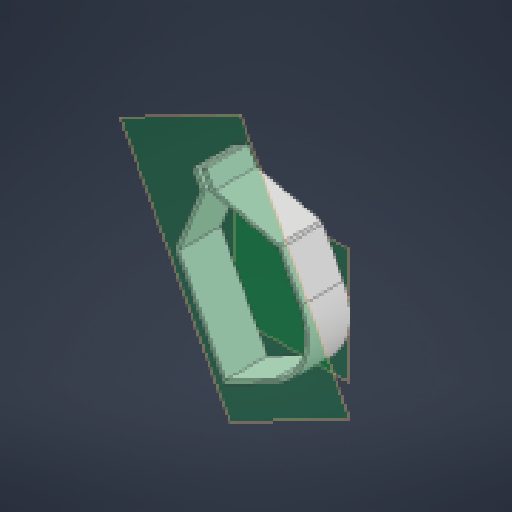
# Autodesk Inventor part: housing_spool
Saved by Autodesk Inventor 2024 (Build 280153000, 153)
## iProperties
Created: 2026-03-24
Part Number: housing_spool
Material: Generic
Document SubType Name: Modeling
Designer: schar
Density: 1 g/cm^3
Appearance: Default
Author: schar
Autodesk Inventor part; units mm, degrees
ref_plane "YZ Plane" through (0, 0, 0) normal (1, 0, 0) x (0, 1, 0)
ref_plane "XZ Plane" through (0, 0, 0) normal (0, 1, 0) x (-1, 0, 0)
ref_plane "XY Plane" through (0, 0, 0) normal (0, 0, 1) x (1, 0, 0)
sketch "Sketch1" plane through (0, 0, 0) normal (0, 0, 1) x (1, 0, 0)
  circle A0 centre (0, 0) radius 30
  line L0 (10.4876, 34.2087) -> (33.8038, -10.3608)
  line L1 (0, 0) -> (41.4605, 21.6898)
  line L2 (0, 0) -> (-43.0442, -22.5183)
  line L3 (-26.5822, -13.9063) -> (-28.3544, -14.8334)
  line L4 (26.5822, 13.9063) -> (28.3544, 14.8334)
  line L5 (8.7104, 28.7647) -> (-22.4507, 46.1509)
  line L6 (-16.4978, 49.2651) -> (10.4876, 34.2087)
  line L7 (-25.1089, 44.7603) -> (-28.5964, 9.2479)
  line L8 (-34.082, 10.8925) -> (-31.0618, 41.6461)
  circle A1 centre (0, 0) radius 32
  circle A2 centre (0, 0) radius 34
  line L9 (15.7605, -30.1265) -> (-26.153, -52.0533)
  line L10 (-30.1265, -15.7605) -> (-6.3352, -61.238)
  line L11 (-30.1265, -15.7605) -> (-49.9852, 22.1997)
  line L12 (-10.7657, -33.6771) -> (-34.082, 10.8925)
  line L13 (10.4876, 34.2087) -> (-34.082, 10.8925)
  line L14 (-34.082, 10.8925) -> (-52.6736, 1.1664)
  line L15 (10.4876, 34.2087) -> (31.4936, 45.1979)
  line L16 (30.1265, 15.7605) -> (13.2261, 48.0659)
  line L17 (28.3544, 14.8334) -> (11.454, 47.1389)
  line L18 (-28.3544, -14.8334) -> (-48.1167, 22.9426)
  line L19 (14.8334, -28.3544) -> (-13.521, -43.1878)
  line L20 (16.5572, 37.384) -> (-22.4507, 46.1509)
  line L21 (-22.4507, 46.1509) -> (-20.6785, 47.078)
  line L22 (16.5572, 37.384) -> (20.2036, 53.6084)
  line L23 (16.5572, 37.384) -> (16.9957, 39.3353)
  line L24 (16.9957, 39.3353) -> (-19.7098, 47.5848)
  line L25 (-19.7098, 47.5848) -> (-20.6785, 47.078)
  line L26 (18.3293, 38.3111) -> (16.9957, 39.3353)
  line L27 (-61.7786, 118.0912) -> (-13.9743, 26.7122)
  line L28 (-42.0046, 8.4697) -> (-27.8498, 43.3264)
  line L29 (-40.1516, 7.7172) -> (-25.1089, 44.7603)
  line L30 (-25.1089, 44.7603) -> (-26.8811, 43.8332)
  line L31 (-27.8498, 43.3264) -> (-26.8811, 43.8332)
  line L32 (-40.1516, 7.7172) -> (-42.0046, 8.4697)
  line L33 (-41.9237, 6.7901) -> (-42.0046, 8.4697)
  line L34 (-40.1516, 7.7172) -> (-55.5588, 13.9738)
  line L35 (-19.7098, 47.5848) -> (-24.3452, 56.4455)
  line L36 (-21.1333, 58.1259) -> (-27.0861, 55.0117)
  line L37 (-22.4507, 46.1509) -> (-27.0861, 55.0117)
  line L38 (-27.0861, 55.0117) -> (-24.3452, 56.4455)
  line L39 (-25.1089, 44.7603) -> (-29.7443, 53.621)
  line L40 (-29.7443, 53.621) -> (-35.6972, 50.5068)
  line L41 (-25.1089, 44.7603) -> (-29.7443, 53.621)
  line L42 (-27.8498, 43.3264) -> (-32.4852, 52.1871)
  line L43 (-29.7443, 53.621) -> (-32.4852, 52.1871)
  line L44 (-13.521, -43.1878) -> (-28.3544, -14.8334)
  line L45 (-61.8482, 118.2241) -> (-14.0438, 26.8451)
  point P0 (8.2214, 9.3684)
  point P1 (-61.7786, 118.0912)
  point P2 (-13.9743, 26.7122)
  point P3 (-14.366, -45.887)
  dimension "d0" = 2
  dimension "d1" = 2
  dimension "d2" = 68
  dimension "d3" = 34
  dimension "d4" = 2
  dimension "d5" = 2
  dimension "d44" = 64
  dimension "d45" = 49.717
  dimension "d46" = 73.507
  dimension "d47" = 7.058
  dimension "d48" = 25.45
  dimension "d49" = 35.85
  dimension "d50" = 25.85
  dimension "d51" = 8.85
  dimension "d52" = 34
  dimension "d53" = 59.15
  dimension "d54" = 12.6858
  dimension "d55" = 11.008
  dimension "d56" = 2.5291
  dimension "d57" = 9.7185
  dimension "d58" = 5.4088
  dimension "d59" = 107.8247
  dimension "d60" = 12.9217
  dimension "d61" = 13.4301
  dimension "d62" = 8.3223
  dimension "d63" = 25.85
  dimension "d64" = 76.7748
  dimension "d65" = 27.2963
  dimension "d66" = 23.2359
  dimension "d67" = 27.4483
  dimension "d68" = 27.4398
  dimension "d69" = 37.885
  dimension "d70" = 55.2569
  dimension "d71" = 57.4671
  dimension "d72" = 11.0758
  dimension "d73" = 75.18
  dimension "d74" = 84.0044
  dimension "d75" = 19.73
  dimension "d76" = -20.9599
  constraints: 90 end point, 14 point on line, 11 parallel, 8 collinear, 7 perpendicular, 7 point on circle, 5 tangent, 3 centre point, 2 coincident, 14 other
  measures "d0" distance of L3.start L18.start
  measures "d1" distance of L4.start L4.end
  measures "d2" diameter of A2
  measures "d3" distance between parallel lines of L2 L9
  measures "d4" distance of L5.end L25.end
  measures "d5" distance of L20.start L23.end
  measures "d44" diameter of A1
  measures "d45" angle of L34 L14
  measures "d46" angle of L32 L8
  measures "d47" angle of L5 L34
  measures "d48" distance between parallel lines of L2 L14
  measures "d49" distance between parallel lines of L43 L14
  measures "d50" distance between parallel lines of L31 L14
  measures "d51" distance between parallel lines of L11 L12
  measures "d52" distance of the line from the sketch origin of L11
  measures "d53" distance between parallel lines of L0 L11
  measures "d54" distance from line of L34.end L14
  measures "d55" distance from line of L14.end L33
  measures "d56" distance from line of L2.end L33
  measures "d57" distance from line of L11.end L34
  measures "d58" distance from line of L18.end L33
  measures "d59" distance from line of point (-61.779, 118.091) L14
  measures "d60" distance from line of L9.end L33
  measures "d61" distance from line of L7.end L33
  measures "d62" distance from line of L40.end L33
  measures "d63" distance from line of L8.end L14
  measures "d64" distance from line of L10.end L14
  measures "d65" distance from line of L12.start L34
  measures "d66" distance from line of L36.start L33
  measures "d67" distance from line of point (-13.974, 26.712) L34
  measures "d68" distance from line of L6.start L33
  measures "d69" distance from line of L5.start L34
  measures "d70" distance from line of L17.end L33
  measures "d71" distance from line of L16.end L32
  measures "d72" distance from line of L0.end L34
  measures "d73" distance from line of L15.end L33
  measures "d74" distance from line of L1.end L33
  measures "d75" distance from line of point (8.221, 9.368) L34
  measures "d76" distance from line of point (8.221, 9.368) L14
ref_plane "Work Plane1" through (0, 0, -14) normal (0, 0, -1) x (-1, 0, 0)
extrude "Extrusion1" add sketch "Sketch1" against normal up to surface (14 mm away) contours L17 A2 L1 | L1 A2 L0 A1 | L0 A2 L19 A1 | A2 L17 L15 L16 | L15 L22 L26 | L20 L6 L24 L17 | L17 L24 L22 | L44 A2 L2 | L2 A2 L18 | L9 L10 A2 L44 L19 | L20 L21 L25 L24 L6 | L11 L14 L18 A2 | L37 L36 L35 L25 L21 | L33 L32 L14 | L32 L28 L18 | L18 L28 L8 L29 | L8 L28 L31 L30 L29 | L30 L31 L42 L40 L39
ref_plane "Work Plane2" through (-8.5115, 15.9463, 10) normal (0, 0, -1) x (-0.886074, -0.4635438, 0)
sketch "Sketch3" plane through (0, 0, 0) normal (0, 0, 1) x (1, 0, 0)
  line L0 (-29.7443, 53.621) -> (-32.4852, 52.1871) projected
  line L1 (-32.4852, 52.1871) -> (-27.8498, 43.3264) projected
  line L2 (-27.8498, 43.3264) -> (-42.0046, 8.4697) projected
  line L3 (-42.0046, 8.4697) -> (-41.9237, 6.7901) projected
  line L4 (-41.9237, 6.7901) -> (-14.366, -45.887) projected
  line L5 (-14.366, -45.887) -> (15.7605, -30.1265) projected
  arc A0 (15.7605, -30.1265) -> (30.1265, 15.7605) centre (0, 0) ccw projected
  line L6 (30.1265, 15.7605) -> (18.3293, 38.3111) projected
  line L7 (18.3293, 38.3111) -> (16.9957, 39.3353) projected
  line L8 (16.9957, 39.3353) -> (-19.7098, 47.5848) projected
  line L9 (-19.7098, 47.5848) -> (-24.3452, 56.4455) projected
  line L10 (-24.3452, 56.4455) -> (-27.0861, 55.0117) projected
  line L11 (-27.0861, 55.0117) -> (-22.4507, 46.1509) projected
  line L12 (-22.4507, 46.1509) -> (16.5572, 37.384) projected
  line L13 (16.5572, 37.384) -> (28.3544, 14.8334) projected
  arc A1 (14.8334, -28.3544) -> (28.3544, 14.8334) centre (0, 0) ccw projected
  line L14 (14.8334, -28.3544) -> (-13.521, -43.1878) projected
  line L15 (-13.521, -43.1878) -> (-40.1516, 7.7172) projected
  line L16 (-40.1516, 7.7172) -> (-25.1089, 44.7603) projected
  line L17 (-25.1089, 44.7603) -> (-29.7443, 53.621) projected
extrude "Extrusion2" add sketch "Sketch3" along normal up to surface (10 mm away)
sketch "Sketch4" plane through (-14.366, -45.887, 10) normal (0, 0, 1) x (0.886074, 0.4635438, 0)
  line L0 (8.7, 9) -> (-10.15, 9) projected
  line L1 (-10.15, 19) -> (-10.15, 9) projected
  line L2 (-10.15, 9) -> (8.7, 9) projected
  line L3 (8.7, 19) -> (8.7, 9) projected
  line L4 (8.7, 19) -> (-10.15, 19) projected
  circle A0 centre (-5.15, 14) radius 2.5 projected
  line L5 (8.7, 59.3) -> (-10.15, 59.3) projected
  line L6 (-10.15, 59.3) -> (-10.15, 49.3) projected
  line L7 (-10.15, 49.3) -> (8.7, 49.3) projected
  line L8 (8.7, 59.3) -> (8.7, 49.3) projected
  circle A1 centre (-5.15, 54.3) radius 2.5 projected
  line L9 (59, 49.3) -> (59, 59.3) projected
  line L10 (59, 49.3) -> (77.85, 49.3) projected
  line L11 (77.85, 49.3) -> (77.85, 59.3) projected
  line L12 (77.85, 59.3) -> (59, 59.3) projected
  circle A2 centre (72.85, 54.3) radius 2.5 projected
  line L13 (59, 9) -> (77.85, 9) projected
  line L14 (77.85, 9) -> (77.85, 19) projected
  line L15 (77.85, 19) -> (59, 19) projected
  line L16 (59, 9) -> (59, 19) projected
  circle A3 centre (72.85, 14) radius 2.5 projected
  line L17 (12.7, 24.85) -> (8.7, 24.85) projected
  line L18 (8.7, 24.85) -> (8.7, 9) projected
  line L19 (8.7, 9) -> (59, 9) projected
  line L20 (59, 9) -> (59, 59.3) projected
  line L21 (59, 59.3) -> (42.0682, 85.15) projected
  line L22 (42.0682, 85.15) -> (42.0682, 95.15) projected
  line L23 (42.0682, 95.15) -> (35.35, 95.15) projected
  line L24 (35.35, 95.15) -> (35.35, 85.15) projected
  line L25 (35.35, 85.15) -> (54.9017, 55.3) projected
  line L26 (54.9017, 55.3) -> (55, 55.3) projected
  line L27 (55, 55.3) -> (55, 13) projected
  line L28 (55, 13) -> (12.7, 13) projected
  line L29 (12.7, 13) -> (12.7, 24.85) projected
  line L30 (77.85, 9) -> (59, 9) projected
  line L31 (59, 9) -> (59, 7) projected
  line L32 (77.85, 7) -> (59, 7) projected
  line L33 (77.85, 9) -> (77.85, 7) projected
  line L34 (8.7, 9) -> (59, 9) projected
  line L35 (8.7, 9) -> (8.7, 7) projected
  line L36 (59, 7) -> (8.7, 7) projected
  line L37 (59, 9) -> (59, 7) projected
  line L38 (59, 19) -> (77.85, 19) projected
  line L39 (77.85, 19) -> (77.85, 21) projected
  line L40 (59, 21) -> (77.85, 21) projected
  line L41 (59, 19) -> (59, 21) projected
  arc A4 (34, 2) -> (66, 34) centre (34, 34) ccw projected
  line L42 (66, 59.45) -> (66, 34) projected
  line L43 (2, 2) -> (2, 59.45) projected
  point P0 (34, 34)
  point P1 (2, 49.3)
  point P2 (2, 59.3)
  point P3 (66, 59.3)
  point P4 (66, 49.3)
  point P5 (62.2666, 19)
  point P6 (53.975, 9)
  point P7 (2, 9)
  point P8 (2, 19)
extrude "Extrusion3" add sketch "Sketch4" against normal blind 3 contours L0 L1 L4 L43 | A4 L16 L19 | L16 A4 L15 L14 L13 | L42 L12 L11 L10 | L43 L7 L6 L5
sketch "Sketch5" plane through (-37.2187, -2.2036, 7) normal (0.4635438, -0.886074, 0) x (0.886074, 0.4635438, 0)
  line L0 (-10.15, 0) -> (0, 0) projected
  line L1 (0, 0) -> (0, -10)
  line L2 (0, -21) -> (0, 3) projected
  line L3 (68, 0) -> (77.85, 0) projected
  line L4 (0, -10) -> (-10.15, 0)
  line L5 (-10.15, 0) -> (68, 0)
  line L6 (68, 0) -> (68, -10)
  line L7 (68, -21) -> (68, 3) projected
  line L8 (68, -10) -> (77.85, 0)
  line L9 (77.85, 3) -> (77.85, 0) projected
  line L10 (-10.15, 3) -> (77.85, 3) projected
  line L11 (-10.15, 3) -> (-10.15, 0) projected
  line L12 (-2.65, 0) -> (-7.65, 0) projected
  point P0 (34, -7)
  dimension "d90" = 10
  dimension "d91" = 10
  constraints: 10 end point, 2 point on line, 1 coincident, 1 horizontal
  measures "d90" distance of L0.end L1.end
  measures "d91" distance of L3.start L6.end
extrude "Extrusion4" add sketch "Sketch5" along normal blind 2 contours L11 L10 L2 L0 | L0 L1 L4 | L7 L10 L9 L3 | L3 L8 L6
sketch "Sketch6" plane through (-41.8542, 6.6572, 10) normal (-0.4635438, 0.886074, 0) x (0.886074, 0.4635438, 0)
  line L0 (0, 0) -> (-10.15, 0) projected
  line L1 (-10.15, 3) -> (0, 13) projected
  line L2 (0, 0) -> (0, 13)
  line L3 (0, 13) -> (-10.15, 3)
  line L4 (-10.15, 3) -> (-10.15, 0)
  line L5 (-10.15, 0) -> (0, 0)
  line L6 (57.0434, 0) -> (77.85, 0) projected
  line L7 (68, 0) -> (68, 3) projected
  line L8 (77.85, 0) -> (68, 0)
  line L9 (68, 13) -> (77.85, 3) projected
  line L10 (68, 0) -> (68, 13)
  line L11 (68, 13) -> (77.85, 3)
  line L12 (77.85, 3) -> (77.85, 0)
  point P0 (34, 10)
  point P1 (68, 3)
  constraints: 16 end point, 2 collinear, 2 parallel, 2 perpendicular, 1 horizontal, 1 vertical
extrude "Extrusion5" add sketch "Sketch6" along normal blind 2
sketch "Sketch7" plane through (-23.1734, -29.0516, 10) normal (-0.4635438, 0.886074, 0) x (0.886074, 0.4635438, 0)
  line L0 (0, 3) -> (-10.15, 3) projected
  line L1 (0, 3) -> (0, 13)
  line L2 (0, 24) -> (0, 0) projected
  line L3 (0, 13) -> (-10.15, 3)
  line L4 (-10.15, 0) -> (0, 0) projected
  line L5 (-10.15, 3) -> (-10.15, 0)
  line L6 (-10.15, 0) -> (0, 0)
  line L7 (0, 0) -> (0, 3)
  line L8 (64.5123, 3) -> (64.5123, 13)
  line L9 (77.85, 0) -> (77.85, 3) projected
  line L10 (64.5123, 13) -> (77.85, 3)
  line L11 (77.85, 3) -> (77.85, 0)
  line L12 (77.85, 0) -> (64.5123, 0)
  line L13 (64.5123, 0) -> (64.5123, 3)
  point P0 (34, 10)
  dimension "d96" = 10
  dimension "d97" = 10
  constraints: 20 end point, 3 collinear, 2 perpendicular, 2 point on line, 1 parallel, 1 vertical
  measures "d96" distance of L0.start L1.end
  measures "d97" distance of L8.start L8.end
extrude "Extrusion6" add sketch "Sketch7" along normal blind 2
sketch "Sketch8" plane through (-18.5379, -37.9123, 7) normal (0.4635438, -0.886074, 0) x (0.886074, 0.4635438, 0)
  line L0 (64.5123, -10) -> (65.4166, -9.322) projected
  line L1 (64.5123, -10) -> (64.5123, 3)
  line L2 (34, 3) -> (66, 3) projected
  line L3 (77.85, 3) -> (68, 3) projected
  line L4 (77.85, 0) -> (57.0434, 0) projected
  line L5 (77.85, 3) -> (77.85, 0)
  line L6 (77.85, 0) -> (64.5123, -10)
  line L7 (0, 3) -> (0, -10) projected
  line L8 (0, -10) -> (0, 3)
  line L9 (-10.15, 3) -> (-10.15, 0) projected
  line L10 (0, 3) -> (-10.15, 3)
  line L11 (-10.15, 3) -> (-10.15, 0)
  line L12 (-10.15, 0) -> (0, -10)
  line L13 (-10.15, 3) -> (77.85, 3) projected
  point P0 (34, -7)
  point P1 (65.4166, -9.322)
  constraints: 14 end point, 3 vertical, 2 perpendicular, 1 point on line
extrude "Extrusion7" add sketch "Sketch8" along normal blind 2
sketch "Sketch9" plane through (18.3293, 38.3111, -3) normal (-0.886074, -0.4635438, 0) x (0, 0, 1)
  line L0 (10, -0.15) -> (0, -0.15) projected
  line L1 (10, -0.15) -> (13, -0.15)
  line L2 (13, -12.15) -> (13, 1.85) projected
  line L3 (10, 1.85) -> (0, 1.85) projected
  line L4 (0, 1.85) -> (13, 1.85)
  line L5 (13, 1.85) -> (13, -0.15)
  line L6 (13, -0.15) -> (0, -0.15)
  line L7 (0, -0.15) -> (0, 1.85)
  point P0 (3, -25.45)
  point P1 (13, 1.85)
  constraints: 10 end point, 2 horizontal, 2 parallel, 1 perpendicular, 1 point on line
extrude "Extrusion8" add sketch "Sketch9" along normal up to surface surface through (16.5572, 37.384, 0) normal (-0.2192779, -0.9756624, 0)
sketch "Sketch10" plane through (38.6247, -8.0081, -3) normal (-0.886074, -0.4635438, 0) x (0, 0, 1)
  line L0 (0, 0) -> (10, 0) projected
  line L1 (13, -2) -> (13, 12) projected
  line L2 (0, -2) -> (13, -2)
  line L3 (13, -2) -> (13, 0)
  line L4 (13, 0) -> (0, 0)
  line L5 (0, 0) -> (0, -2)
  point P0 (3, 25)
  constraints: 8 end point, 2 parallel, 1 horizontal, 1 perpendicular, 1 point on line
extrude "Extrusion9" add sketch "Sketch10" along normal up to surface round surface about axis through (0, 0, 0) along (0, 0, -1) radius 34 far side no
sketch "Sketch11" plane through (-41.9237, 6.7901, 10) normal (0.886074, 0.4635438, 0) x (0, 0, -1)
  line L0 (13, 1.85) -> (3, 1.85) projected
  line L1 (0, 1.85) -> (0, -12.15) projected
  line L2 (13, 1.85) -> (0, 1.85)
  line L3 (0, 1.85) -> (0, -0.15)
  line L4 (13, -0.15) -> (3, -0.15) projected
  line L5 (0, -0.15) -> (13, -0.15)
  line L6 (13, -0.15) -> (13, 1.85)
  point P0 (10, -25.45)
  point P1 (0, -0.15)
  point P2 (3, -0.15)
  constraints: 8 end point, 3 perpendicular, 1 horizontal
extrude "Extrusion10" add sketch "Sketch11" along normal up to surface surface through (-25.1089, 44.7603, 0) normal (0.9265198, -0.3762459, 0)
sketch "Sketch12" plane through (15.7605, -30.1265, -14) normal (0.4635438, -0.886074, 0) x (0.886074, 0.4635438, 0)
  line L0 (6.5, 3.5) -> (-6.5, 3.5) projected
  line L1 (-6.5, 10.5) -> (6.5, 10.5) projected
  line L2 (-6.5, 3.5) -> (-6.5, 10.5)
  circle A0 centre (-6.5, 7) radius 2.5
  point P0 (0, 14)
  dimension "d108" = 5
  constraints: 2 end point, 1 centre point, 1 midpoint, 1 perpendicular
  measures "d108" diameter of A0
extrude "Extrusion11" cut sketch "Sketch12" against normal up to surface (2 mm away)
body "Solid1"
